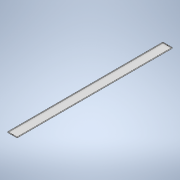
# Autodesk Inventor part: dwc
Saved by Autodesk Inventor 2020 (Build 240168000, 168)
## iProperties
Created: 2019-09-26
Part Number: dwc
Material: Generic
Document SubType Name: Modeling
Designer: Abbas
Density: 1 g/cm^3
Appearance: Default
Author: Abbas
Autodesk Inventor part; units mm, degrees
ref_plane "YZ Plane" through (0, 0, 0) normal (1, 0, 0) x (0, 1, 0)
ref_plane "XZ Plane" through (0, 0, 0) normal (0, 1, 0) x (-1, 0, 0)
ref_plane "XY Plane" through (0, 0, 0) normal (0, 0, 1) x (1, 0, 0)
sketch "Sketch1" plane through (0, 0, 0) normal (0, 1, 0) x (-1, 0, 0)
  line L0 (47005.8752, -47004.4138) -> (50005.8752, -47004.4138)
  line L1 (50005.8752, -47004.4138) -> (50005.8752, 2995.5862)
  line L2 (50005.8752, 2995.5862) -> (47005.8752, 2995.5862)
  line L3 (47005.8752, 2995.5862) -> (47005.8752, -47004.4138)
  point P0 (0, 0)
  dimension "d0" = 3000
  dimension "d1" = 50000
  constraints: 8 end point, 2 parallel, 1 horizontal, 1 perpendicular
  measures "d0" distance of L2.end L1.end
  measures "d1" distance of L1.end L0.end
extrude "Extrusion1" add sketch "Sketch1" along normal blind 300
sketch "Sketch2" plane through (0, 300, 0) normal (0, 1, 0) x (1, 0, 0)
  line L0 (-47025.8752, 46984.4138) -> (-49985.8752, 46984.4138)
  line L1 (-49985.8752, 46984.4138) -> (-49985.8752, -2975.5862)
  line L2 (-49985.8752, -2975.5862) -> (-47025.8752, -2975.5862)
  line L3 (-47025.8752, -2975.5862) -> (-47025.8752, 46984.4138)
  line L4 (-47005.8752, -2995.5862) -> (-47005.8752, 47004.4138) projected
  line L5 (-50005.8752, 47004.4138) -> (-50005.8752, -2995.5862) projected
  line L6 (-47005.8752, 47004.4138) -> (-50005.8752, 47004.4138) projected
  line L7 (-50005.8752, -2995.5862) -> (-47005.8752, -2995.5862) projected
  point P0 (0, 0)
  dimension "d4" = 20
  dimension "d5" = 20
  dimension "d6" = 20
  dimension "d7" = 20
  constraints: 8 end point, 2 parallel, 1 horizontal, 1 perpendicular
  measures "d4" distance between parallel lines of L4 L3
  measures "d5" distance between parallel lines of L5 L1
  measures "d6" distance between parallel lines of L6 L0
  measures "d7" distance between parallel lines of L7 L2
extrude "Extrusion2" cut sketch "Sketch2" against normal blind 280 contours L3 L2 L1 L0
sketch "Sketch3" plane through (-50005.8752, 0, 2995.5862) normal (0, 0, 1) x (1, 0, 0)
  line L0 (2980, 300) -> (20, 300) projected
  circle A0 centre (1500, 150) radius 75
  point P0 (50005.8752, 0)
  dimension "d10" = 150
  constraints: 1 centre point
  measures "d10" diameter of A0
extrude "Extrusion3" cut sketch "Sketch3" against normal blind 55000
body "Solid1"
